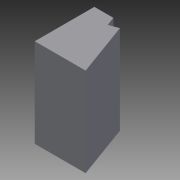
# Autodesk Inventor part: rigid connector
Saved by Autodesk Inventor 2015 (Build 190159000, 159)
## iProperties
Created: 2014-07-29
Part Number: rigid connector
Material: Generic
Document SubType Name: Modeling
Designer: Nick
Density: 1 g/cm^3
Appearance: Default
Author: Nick
Autodesk Inventor part; units mm, degrees
ref_plane "YZ Plane" through (0, 0, 0) normal (1, 0, 0) x (0, 1, 0)
ref_plane "XZ Plane" through (0, 0, 0) normal (0, 1, 0) x (-1, 0, 0)
ref_plane "XY Plane" through (0, 0, 0) normal (0, 0, 1) x (1, 0, 0)
sketch "Sketch1" plane through (0, 0, 0) normal (0, 0, 1) x (1, 0, 0)
  line L0 (-5.5771, -0.1491) -> (-6.9867, -0.6621)
  line L1 (-6.9867, -0.6621) -> (-7.4997, 0.7474)
  line L2 (-2.4841, -8.6471) -> (-10.4997, -8.6471)
  line L3 (-10.4997, -8.6471) -> (-10.4997, 0.7474)
  line L4 (-10.4997, 0.7474) -> (-7.4997, 0.7474)
  line L5 (-2.4841, -8.6471) -> (-5.5771, -0.1491)
  dimension "d8" = 3
  dimension "d10" = 70
  dimension "d11" = 8.498
  dimension "d12" = 1.5
  dimension "d13" = 1.5
  constraints: 12 end point, 2 parallel, 2 perpendicular, 1 vertical
  measures "d8" distance of L3.end L1.end
  measures "d10" angle of L2 L5
  measures "d11" vertical distance of L2.start L0.start
  measures "d12" distance of L0.start L0.end
  measures "d13" distance of L0.end L1.end
extrude "Extrusion1" add sketch "Sketch1" along normal blind 14
body "Solid1"
